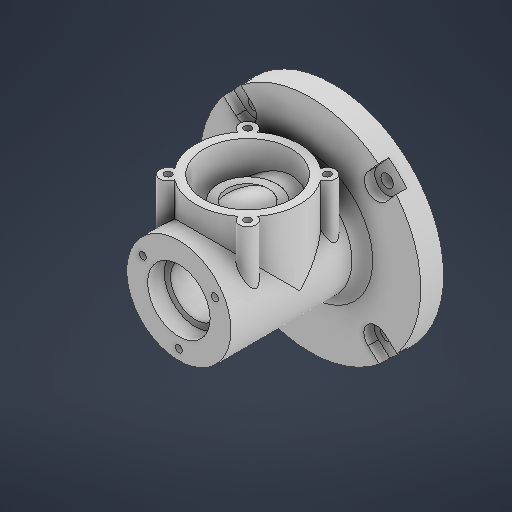
# Autodesk Inventor part: 12
Saved by Autodesk Inventor 2026.2 (Build 302298010, 298A)
## iProperties
Created: 2026-03-11
Part Number: 12
Material: Generico
Document SubType Name: Modeling
Designer: mahsa
Density: 1 g/cm^3
Appearance: Default
Author: mahsa
Autodesk Inventor part; units mm, degrees
sketch "Schizzo1" plane through (0, 0, 0) normal (0, 0, 1) x (1, 0, 0)
  circle A0 centre (0, 0) radius 25
  circle A1 centre (0, 0) radius 15
  dimension "d0" = 50
  dimension "d1" = 30
  constraints: 2 centre point, 2 coincident
  measures "d0" diameter of A0
  measures "d1" diameter of A1
extrude "Estrusione1" add sketch "Schizzo1" against normal blind 10
sketch "Schizzo2" plane through (0, 0, 0) normal (0, 0, 1) x (1, 0, 0)
  circle A0 centre (0, 0) radius 12
  circle A1 centre (0, 0) radius 25
  dimension "d4" = 24
  dimension "d5" = 50
  constraints: 2 centre point, 2 coincident
  measures "d4" diameter of A0
  measures "d5" diameter of A1
extrude "Estrusione2" add sketch "Schizzo2" along normal blind 45
sketch "Schizzo3" plane through (0, 0, 45) normal (0, 0, 1) x (1, 0, 0)
  circle A0 centre (0, 0) radius 15
  circle A1 centre (0, 0) radius 25
  dimension "d8" = 30
  dimension "d9" = 50
  constraints: 2 centre point, 2 coincident
  measures "d8" diameter of A0
  measures "d9" diameter of A1
extrude "Estrusione3" add sketch "Schizzo3" along normal blind 8
ref_plane "Piano di lavoro1" through (0, 36, 0) normal (0, 1, 0) x (-1, 0, 0)
sketch "Schizzo5" plane through (0, 36, 0) normal (0, 1, 0) x (-1, 0, 0)
  line L0 (-25, -10) -> (25, -10) projected
  line L1 (0, -10) -> (0, 20)
  circle A0 centre (0, 20) radius 21
  circle A1 centre (0, 20) radius 25
  line L2 (0, 20) -> (33.741, 20) construction
  circle A2 centre (19.0919, 0.9081) radius 4
  circle A3 centre (19.0919, 39.0919) radius 4
  circle A4 centre (-19.0919, 39.0919) radius 4
  circle A5 centre (-19.0919, 0.9081) radius 4
  point P0 (0, 0)
  point P1 (15.1688, 0.1277)
  point P2 (19.8723, 4.8312)
  point P3 (19.8723, 35.1688)
  point P4 (15.1688, 39.8723)
  point P5 (-15.1688, 39.8723)
  point P6 (-19.8723, 35.1688)
  point P7 (-19.8723, 4.8312)
  point P8 (-15.1688, 0.1277)
  dimension "d18" = 30
  dimension "d19" = 42
  dimension "d26" = 50
  dimension "d29" = 8
  dimension "d32" = 360
  dimension "d34" = 38.1838
  constraints: 6 centre point, 4 coincident, 4 end point, 1 horizontal, 1 midpoint, 1 vertical, 9 other
  measures "d18" distance of L1.start L1.end
  measures "d19" diameter of A0
  measures "d26" diameter of A1
  measures "d29" diameter of A2
  measures "d34" distance of A3.centre A4.centre
extrude "Estrusione5" add sketch "Schizzo5" against normal up to surface
ref_plane "Piano di lavoro2" through (0, 25, 0) normal (0, 1, 0) x (-1, 0, 0)
sketch "Schizzo6" plane through (0, 25, 0) normal (0, 1, 0) x (-1, 0, 0)
  circle A0 centre (0, 20) radius 21 projected
  circle A1 centre (0, 20) radius 10
  circle A2 centre (0, 20) radius 14
  point P0 (0, 0)
  dimension "d38" = 20
  dimension "d39" = 28
  constraints: 2 centre point, 2 coincident
  measures "d38" diameter of A1
  measures "d39" diameter of A2
extrude "Estrusione6" add sketch "Schizzo6" against normal up to surface contours A2
sketch "Schizzo7" plane through (0, 36, 0) normal (0, 1, 0) x (1, 0, 0)
  arc A0 (15.1688, -39.8723) -> (19.8723, -35.1688) centre (19.0919, -39.0919) ccw projected
  arc A1 (-19.8723, -35.1688) -> (-15.1688, -39.8723) centre (-19.0919, -39.0919) ccw projected
  arc A2 (-15.1688, -0.1277) -> (-19.8723, -4.8312) centre (-19.0919, -0.9081) ccw projected
  arc A3 (19.8723, -4.8312) -> (15.1688, -0.1277) centre (19.0919, -0.9081) ccw projected
  point P0 (0, 0)
  constraints: 4 coincident
hole "Foro1" at (19.0919, 36, 39.0919) at (-19.0919, 36, 39.0919) at (-19.0919, 36, 0.9081) at (19.0919, 36, 0.9081) direction (0, -1, 0) diameter 3.4587 depth 10.8 tip angle 118 thread size "M4x0.5" class "6H" standard "ISO Metric profile"
ref_plane "Piano di lavoro3" through (0, 0, -21) normal (0, 0, -1) x (-1, 0, 0)
sketch "Schizzo8" plane through (0, 0, -21) normal (0, 0, -1) x (-1, 0, 0)
  circle A0 centre (0, 0) radius 53
  circle A1 centre (0, 0) radius 15 projected
  circle A2 centre (0, 0) radius 43
  line L0 (0, 0) -> (68.644, 0)
  line L1 (0, 0) -> (47.762, 0) construction
  arc A3 (36.4365, -27.7377) -> (27.4331, -35.6711) centre (31.9348, -31.7044) ccw
  circle A4 centre (31.9348, -31.7044) radius 3
  line L2 (36.4365, -27.7377) -> (41.2827, -33.2376)
  line L3 (27.4331, -35.6711) -> (32.732, -41.6847)
  arc A5 (27.7377, 36.4365) -> (35.6711, 27.4331) centre (31.7044, 31.9348) ccw
  circle A6 centre (31.7044, 31.9348) radius 3
  line L4 (27.7377, 36.4365) -> (33.2376, 41.2827)
  line L5 (35.6711, 27.4331) -> (41.6847, 32.732)
  arc A7 (-36.4365, 27.7377) -> (-27.4331, 35.6711) centre (-31.9348, 31.7044) ccw
  circle A8 centre (-31.9348, 31.7044) radius 3
  line L6 (-36.4365, 27.7377) -> (-41.2827, 33.2376)
  line L7 (-27.4331, 35.6711) -> (-32.732, 41.6847)
  arc A9 (-27.7377, -36.4365) -> (-35.6711, -27.4331) centre (-31.7044, -31.9348) ccw
  circle A10 centre (-31.7044, -31.9348) radius 3
  line L8 (-27.7377, -36.4365) -> (-33.2376, -41.2827)
  line L9 (-35.6711, -27.4331) -> (-41.6847, -32.732)
  arc A11 (27.4331, -35.6711) -> (35.8688, -27.1741) centre (0, 0) ccw
  arc A12 (35.6711, 27.4331) -> (33.7618, 29.7514) centre (0, 0) ccw
  arc A13 (29.5062, 33.9763) -> (27.1741, 35.8688) centre (0, 0) ccw
  arc A14 (-35.6711, -27.4331) -> (-33.7618, -29.7514) centre (0, 0) ccw
  arc A15 (-29.5062, -33.9763) -> (-27.1741, -35.8688) centre (0, 0) ccw
  arc A16 (-27.4331, 35.6711) -> (-29.7514, 33.7618) centre (0, 0) ccw
  arc A17 (-33.9763, 29.5062) -> (-35.8688, 27.1741) centre (0, 0) ccw
  dimension "d50" = 106
  dimension "d52" = 86
  dimension "d57" = 12
  dimension "d58" = 6
  dimension "d61" = 360
  dimension "d63" = 63.6392
  dimension "d64" = 65.9695
  constraints: 38 point on circle, 20 end point, 17 centre point, 8 coincident, 2 horizontal, 2 tangent, 1 point on line, 45 other
  measures "d50" diameter of A0
  measures "d52" diameter of A2
  measures "d57" diameter of A3
  measures "d58" diameter of A4
  measures "d63" vertical distance of A9.centre A7.centre
  measures "d64" vertical distance of L9.end L6.end
extrude "Estrusione7" add sketch "Schizzo8" against normal blind 11 contours L0 A2 A5 L5 A0 | A0 L2 A3 A2 L0 | A2 A3 A9 A7 A5 | L4 A5 A2 A7 L7 A0 | A0 L8 A9 A2 A3 L3 | L6 A7 A2 A9 L9 A0 | A1
sketch "Schizzo9" plane through (0, 0, -10) normal (0, 0, 1) x (1, 0, 0)
  point P0 (0, 0)
extrude "Estrusione8" add sketch "Schizzo8" against normal blind 6 contours L5 A12 A6 A13 A5 L4 A0 | A0 L3 A11 A4 A3 L2 | A5 A2 A6 A12 | A5 A2 A6 | A3 A11 A4 A2 | A2 A4 A3 | L7 A16 A8 A17 A7 L6 A0 | A0 L9 A14 A10 A15 A9 L8 | A3 A2 A4 A11 | A5 A13 A6 A2 | A7 A2 A8 A16 | A7 A2 A8 | A9 A15 A10 A2 | A2 A10 A9 | A9 A2 A10 A14 | A7 A17 A8 A2
fillet "Raccordo faccia1" radius 5 1 edges at (-25, 0, -10)
sketch "Schizzo10" plane through (0, 0, 53) normal (0, 0, 1) x (1, 0, 0)
  circle A0 centre (0, 0) radius 20
  point P0 (0, -20)
  point P1 (0, -20)
  point P2 (17.3205, 10)
  point P3 (-17.3205, 10)
  dimension "d70" = 40
  dimension "d73" = 360
  constraints: 2 coincident, 1 vertical alignment, 6 other
hole "Foro2" at (0, -20, 53) at (17.3205, 10, 53) at (-17.3205, 10, 53) direction (0, 0, -1) diameter 3.4587 depth 12 tip angle 118 thread size "M4x0.5" class "6H" standard "ISO Metric profile"
equation "\"d35\" = d34"
